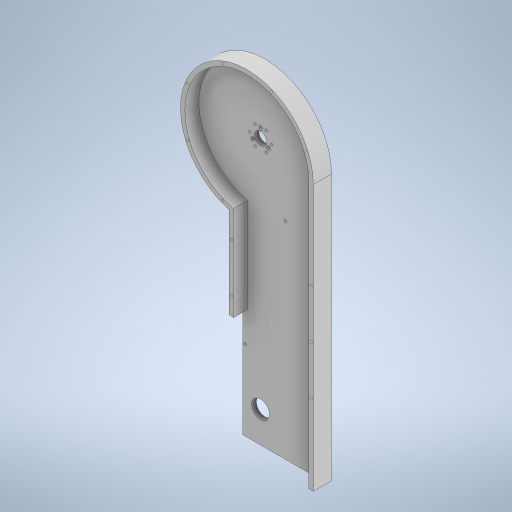
# Autodesk Inventor part: legparts_05(three)
Saved by Autodesk Inventor 2024.3 (Build 283343000, 343)
## iProperties
Created: 2024-10-20
Part Number: legparts_05(three)
Material: 一般
Document SubType Name: Modeling
Designer: 佐藤智貴
Density: 1 g/cm^3
Appearance: 既定
Mass: 230.129 g
Surface Area: 1127.29 cm^2
Volume: 230.129 cm^3
Author: 佐藤智貴
Autodesk Inventor part; units mm, degrees
ref_plane "YZ Plane" through (0, 0, 0) normal (1, 0, 0) x (0, 1, 0)
ref_plane "XZ Plane" through (0, 0, 0) normal (0, 1, 0) x (-1, 0, 0)
ref_plane "XY Plane" through (0, 0, 0) normal (0, 0, 1) x (1, 0, 0)
sketch "スケッチ1" plane through (0, 0, 0) normal (0, 0, 1) x (1, 0, 0)
  circle A0 centre (0, 0) radius 75
  circle A1 centre (0, 0) radius 7
  dimension "d0" = 150
  dimension "d1" = 14
  constraints: 2 centre point, 1 coincident
  measures "d0" diameter of A0
  measures "d1" diameter of A1
extrude "押し出し1" add sketch "スケッチ1" along normal blind 20.5
sketch "スケッチ2" plane through (0, 0, 20.5) normal (0, 0, 1) x (1, 0, 0)
  circle A0 centre (0, 0) radius 72.5
  line L0 (0, 0) -> (0, 93.3217)
  line L1 (0, 0) -> (-34.4548, 83.1811)
  line L2 (0, 0) -> (43.8509, 75.4285)
  point P0 (-27.7445, 66.9813)
  point P1 (-66.9813, 27.7445)
  point P2 (-66.9813, -27.7445)
  point P3 (-27.7445, -66.9813)
  point P4 (27.7445, -66.9813)
  point P5 (66.9813, -27.7445)
  point P6 (66.9813, 27.7445)
  point P7 (27.7445, 66.9813)
  dimension "d4" = 145
  dimension "d5" = 22.5
  dimension "d8" = 360
  constraints: 6 end point, 1 coincident, 1 point on line, 1 vertical, 12 other
  measures "d5" angle of L1 L0
hole "穴1" at (-27.7445, 66.9813, 20.5) at (-66.9813, 27.7445, 20.5) at (-66.9813, -27.7445, 20.5) at (-27.7445, -66.9813, 20.5) at (27.7445, -66.9813, 20.5) at (66.9813, -27.7445, 20.5) at (66.9813, 27.7445, 20.5) at (27.7445, 66.9813, 20.5) direction (0, 0, -1) diameter 2.459 end through all
sketch "スケッチ3" plane through (0, 0, 20.5) normal (0, 0, 1) x (1, 0, 0)
  circle A0 centre (0, 0) radius 70
  dimension "d17" = 140
  constraints: 1 centre point, 1 coincident
  measures "d17" diameter of A0
extrude "押し出し2" cut sketch "スケッチ3" against normal blind 15.5
sketch "スケッチ4" plane through (0, 0, 0) normal (0, 0, -1) x (-1, 0, 0)
  line L0 (0, 0) -> (0, -80.557)
  circle A0 centre (0, 0) radius 75 projected
  line L1 (-75, 0) -> (-75, -300)
  line L2 (75, 0) -> (75, -300)
  line L3 (-75, -300) -> (75, -300)
  line L4 (75, 0) -> (48.7534, -300)
  point P0 (75, 0)
  point P1 (-48.7534, -300)
  point P2 (75, 0)
  point P3 (73.8606, -13.0236)
  point P4 (-48.5, -27.9955)
  point P5 (63.5, -39.9093)
  dimension "d21" = 75
  dimension "d23" = 150
  dimension "d24" = 300
  dimension "d25" = 300
  dimension "d56" = 0
  dimension "d89" = 85
  constraints: 10 end point, 2 point on line, 1 perpendicular, 1 vertical, 2 other
  measures "d21" distance from line of L1 L0.start
  measures "d23" distance between parallel lines of L2 L1
  measures "d24" distance of L2.start L2.end
  measures "d25" distance of L1.start L1.end
  measures "d56" angle of L2 L0
  measures "d89" angle of L3 L4
extrude "押し出し3" add sketch "スケッチ4" against normal blind 5 contours A0 L4 L3 L1
sketch "スケッチ5" plane through (0, 0, 5) normal (0, 0, 1) x (1, 0, 0)
  line L0 (-48.7534, -300) -> (75, -300) projected
  circle A0 centre (0, 0) radius 75 projected
  circle A1 centre (0, 0) radius 70 projected
  line L1 (-48.7534, -300) -> (22.2534, -300)
  circle A2 centre (0, 0) radius 75
  line L2 (75, 0) -> (75, -300)
  line L3 (22.2534, -300) -> (75, -300)
  line L4 (70, -26.9258) -> (70, -295)
  line L5 (-44.1717, -295) -> (70, -295)
  line L6 (0, 0) -> (0, -325.2002)
  line L7 (-15, 0) -> (-15, -325.2002)
  circle A3 centre (0, 0) radius 85
  line L8 (-20, 0) -> (-20, -325.2002)
  point P0 (-75, 0)
  point P1 (13.1233, -300)
  point P2 (0, -300)
  point P3 (58.3325, -334.9093)
  point P4 (-20, -300)
  point P5 (-15, -295)
  point P6 (-15, -73.4847)
  point P7 (-20, -72.2842)
  dimension "d33" = 5
  dimension "d131" = 5
  dimension "d136" = 5
  dimension "d174" = 15
  dimension "d175" = 10
  dimension "d176" = 5
  constraints: 16 end point, 3 parallel, 3 vertical, 2 collinear, 1 centre point, 1 coincident, 1 midpoint, 1 perpendicular, 4 other
  measures "d33" radial gap between concentric circles of A0 A1
  measures "d131" distance between parallel lines of L2 L4
  measures "d136" distance between parallel lines of L0 L5
  measures "d174" distance between parallel lines of L6 L7
  measures "d175" radial gap between concentric circles of A3 A0
  measures "d176" distance between parallel lines of L7 L8
extrude "押し出し4" add sketch "スケッチ5" along normal blind 15.5 contours L0 L6 L5 L4 A3 L2 | L0 L7 L5 L6 | A3 L4 A0 L2 | L0 L8 L5 L7 | L5 L8 A3 L7 | A0 L7 A3 L8
sketch "スケッチ6" plane through (0, 0, 20.5) normal (0, 0, 1) x (1, 0, 0)
  line L0 (-20, -300) -> (75, -300) projected
  arc A0 (75, 0) -> (-20, -72.2842) centre (0, 0) ccw projected
  line L1 (75, -300) -> (75, 0) projected
  line L2 (70, -26.9258) -> (70, -295) projected
  line L3 (-15, -295) -> (-15, -73.4847) projected
  line L4 (-20, -72.2842) -> (-20, -300) projected
  point P0 (72.5, -100)
  point P1 (-17.5, -100)
  point P2 (72.5, -155)
  point P3 (-17.5, -155)
  point P4 (72.5, -210)
  point P5 (-17.5, -210)
  point P6 (13.1233, -300)
  point P7 (-6.5367, 74.7146)
  point P8 (22.2534, -300)
  point P9 (70, -295)
  point P10 (-32.2343, -300)
  dimension "d36" = 375.23
  dimension "d38" = 55
  dimension "d39" = 55
  dimension "d44" = 55
  dimension "d45" = 55
  dimension "d87" = 100
  dimension "d88" = 100
  dimension "d132" = 2.5
  dimension "d133" = 2.5
  dimension "d134" = 2.5
  dimension "d177" = 2.5
  dimension "d178" = 2.5
  dimension "d179" = 2.5
  constraints: 1 point on circle, 1 point on line, 1 other
  measures "d36" distance of point (13.123, -300) point (-6.537, 74.715)
  measures "d38" distance of point (-17.5, -210) point (-17.5, -155)
  measures "d39" distance of point (-17.5, -155) point (-17.5, -100)
  measures "d44" distance of point (72.5, -210) point (72.5, -155)
  measures "d45" distance of point (72.5, -100) point (72.5, -155)
  measures "d87" vertical distance of point (-17.5, -100) point (0, 0)
  measures "d88" vertical distance of point (0, 0) point (72.5, -100)
  measures "d132" distance from line of L1 point (72.5, -100)
  measures "d134" distance from line of L1 point (72.5, -210)
  measures "d177" distance from line of L3 point (-17.5, -100)
  measures "d178" distance from line of L3 point (-17.5, -155)
  measures "d179" distance from line of L4 point (-17.5, -210)
hole "穴2" at (72.5, -100, 20.5) at (-17.5, -100, 20.5) at (72.5, -155, 20.5) at (-17.5, -155, 20.5) at (72.5, -210, 20.5) at (-17.5, -210, 20.5) direction (0, 0, -1) diameter 2.459 end through all
sketch "スケッチ7" plane through (0, 0, 5) normal (0, 0, 1) x (1, 0, 0)
  line L0 (43.5, 0) -> (43.5, -295) projected
  line L1 (43.5, -295) -> (-43.5, -295) projected
  point P0 (0, 0)
  point P1 (0, -265)
  point P2 (75, 0)
  dimension "d57" = 43.5
  dimension "d58" = 30
  measures "d57" distance from line of point (0, -265) L0
  measures "d58" distance from line of L1 point (0, -265)
hole "穴3" at (0, -265, 5) direction (0, 0, -1) diameter 20 end through all
sketch "スケッチ13" plane through (0, 0, 5) normal (0, 0, 1) x (1, 0, 0)
  circle A0 centre (0, 0) radius 43.5
  circle A1 centre (0, 0) radius 12.5
  line L0 (0, 0) -> (-7.2545, 12.5652)
  line L1 (0, 0) -> (0, 17.1386)
  point P0 (-6.25, 10.8253)
  point P1 (-12.5, 0)
  point P2 (-6.25, -10.8253)
  point P3 (6.25, -10.8253)
  point P4 (12.5, 0)
  point P5 (6.25, 10.8253)
  dimension "d110" = 25
  dimension "d107" = 87
  dimension "d111" = 30
  dimension "d112" = 360
  constraints: 4 end point, 2 coincident, 1 centre point, 1 point on line, 1 vertical, 10 other
  measures "d107" diameter of A0
  measures "d111" angle of L1 L0
hole "穴4" at (-6.25, 10.8253, 5) at (6.25, 10.8253, 5) at (12.5, 0, 5) at (6.25, -10.8253, 5) at (-6.25, -10.8253, 5) at (-12.5, 0, 5) direction (0, 0, -1) diameter 2.459 depth 8 tip angle 118
sketch "スケッチ14" plane through (0, 0, 5) normal (0, 0, 1) x (1, 0, 0)
  circle A0 centre (0, 0) radius 10.2
  point P0 (0.0737, 10.1997)
  point P1 (0.0737, 10.1997)
  point P2 (-8.8701, -5.036)
  point P3 (8.7964, -5.1637)
  dimension "d122" = 20.4
  dimension "d123" = 360
  constraints: 3 coincident, 7 other
hole "穴5" at (0.0737, 10.1997, 5) at (8.7964, -5.1637, 5) at (-8.8701, -5.036, 5) direction (0, 0, -1) diameter 4 depth 8 tip angle 118
sketch "スケッチ17" plane through (0, 0, 20.5) normal (0, 0, 1) x (1, 0, 0)
  line L0 (70, -295) -> (70, -26.9258) projected
  circle A0 centre (0, 0) radius 75
  circle A1 centre (0, 0) radius 70 projected
  circle A2 centre (0, 0) radius 70
  line L1 (-44.195, -295) -> (70, -295)
  line L2 (75, -300) -> (-48.7534, -300) projected
  line L3 (70.4374, -300) -> (-48.7534, -300)
  line L4 (70, -295) -> (70, -300)
  circle A3 centre (0, 0) radius 70 projected
  line L5 (70, -26.9258) -> (70, 0)
  line L6 (-20, -72.2842) -> (-20, -300) projected
  line L7 (-20, -175) -> (-15.0426, -175)
  line L8 (-15.0426, -175) -> (-15, -175)
  line L9 (-15, -295) -> (-15, -73.4847) projected
  line L10 (-15, -175) -> (-15, -295)
  line L11 (-15, -295) -> (-20, -295)
  line L12 (-20, -295) -> (-20, -175)
  circle A4 centre (-17.5, -210) radius 1.2295 projected
  line L13 (-20, -72.2842) -> (-20, -67.082)
  line L14 (-15, -73.4847) -> (-15, -68.374)
  line L15 (70, -26.9258) -> (70, 0)
  circle A5 centre (-17.5, -155) radius 1.2295 projected
  point P0 (-44.1717, -295)
  point P1 (75, 0)
  point P2 (70, -26.9258)
  point P3 (70, 0)
  dimension "d183" = 20
  constraints: 24 end point, 6 point on line, 3 collinear, 2 coincident, 2 horizontal, 2 parallel, 2 perpendicular, 2 point on circle, 2 vertical, 1 centre point, 1 horizontal alignment, 1 tangent, 2 other
  measures "d183" distance from line of L7 A5.centre
extrude "押し出し12" cut sketch "スケッチ17" against normal blind 15.5 contours L4 L2 L6 L1 | A0 L14 A1 L5 | L1 L6 L7 L8 L9 | A1 | A4
sketch "スケッチ19" plane through (0, 0, 5) normal (0, 0, 1) x (1, 0, 0)
  circle A0 centre (0, 0) radius 75
  line L0 (-73.8606, -13.0236) -> (-48.7534, -300) projected
  line L1 (-75, 0) -> (-48.7534, -300)
  line L2 (-20, -72.2842) -> (-20, -300) projected
  line L3 (-48.7534, -300) -> (-20, -300)
  line L4 (-20, -300) -> (-20, -72.2842)
  constraints: 6 end point, 2 perpendicular, 1 centre point, 1 coincident, 1 collinear, 1 point on circle
extrude "押し出し13" cut sketch "スケッチ19" against normal blind 15.5 contours L2 L3 L0 A0
equation "\"d21\" = 0.5 * d23"
equation "\"d25\" = d24"
equation "\"d44\" = d43"
equation "\"d45\" = d44"
equation "\"d88\" = d87"
equation "\"d133\" = d132"
equation "\"d134\" = d133"
equation "\"d57\" = 0.5 * d86"
equation "\"d43\" = d37"
equation "\"d37\" = 55"
equation "\"d86\" = 87"
